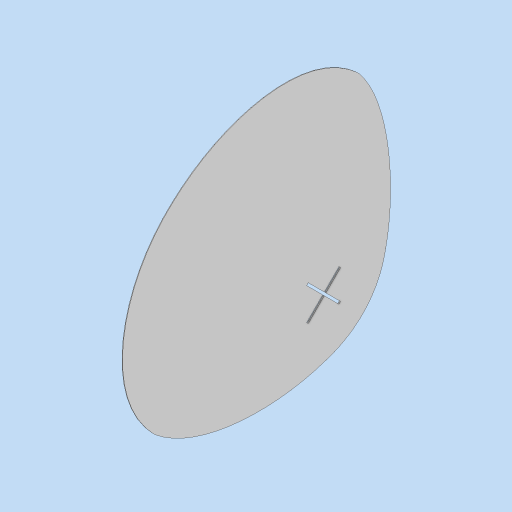
# Autodesk Inventor part: Sticker2
Saved by Autodesk Inventor 2024 (Build 280153000, 153)
## iProperties
Created: 2025-01-25
Part Number: Sticker2
Material: Generic
Document SubType Name: Modeling
Designer: Dmitry
Density: 1 g/cm^3
Appearance: Default
Author: Dmitry
Autodesk Inventor part; units mm, degrees
(part 1 of 3)
ref_plane "YZ Plane" through (0, 0, 0) normal (1, 0, 0) x (0, 1, 0)
ref_plane "XZ Plane" through (0, 0, 0) normal (0, 1, 0) x (-1, 0, 0)
ref_plane "XY Plane" through (0, 0, 0) normal (0, 0, 1) x (1, 0, 0)
sketch "Sketch1" plane through (0, 0, 0) normal (1, 0, 0) x (0, 1, 0)
  line L0 (-21.709644, 35.632021) -> (-25.631404, 35.976699)
  line L1 (-25.631404, 35.976699) -> (-30.886664, 35.950283)
  line L2 (-30.886664, 35.950283) -> (-36.111444, 35.341191)
  line L3 (-59.007004, 23.466691) -> (-59.883304, 22.478631)
  line L4 (-66.774324, 9.489325) -> (-68.001144, 5.643003)
  line L5 (-68.346584, 4.343793) -> (-69.034924, 1.649615)
  line L6 (-69.034924, 1.649615) -> (-70.464944, -6.596495)
  line L7 (-70.464944, -6.596495) -> (-71.331084, -17.731347)
  line L8 (-63.947304, -55.443921) -> (-61.640984, -58.857325)
  line L9 (-61.640984, -58.857325) -> (-60.729124, -59.867433)
  line L10 (-60.729124, -59.867433) -> (-59.807104, -60.803118)
  line L11 (-59.807104, -60.803118) -> (-56.515264, -63.098922)
  line L12 (-56.515264, -63.098922) -> (-51.475904, -65.518755)
  line L13 (-51.475904, -65.518755) -> (-46.101264, -67.289516)
  line L14 (-46.101264, -67.289516) -> (-42.187124, -68.287253)
  line L15 (-42.187124, -68.287253) -> (-40.871404, -68.578007)
  line L16 (-40.871404, -68.578007) -> (-38.123124, -69.126469)
  line L17 (-29.769064, -70.227534) -> (-18.534644, -70.775971)
  line L18 (-18.534644, -70.775971) -> (-7.300224, -70.206858)
  line L19 (1.048756, -69.074094) -> (3.794496, -68.507751)
  line L20 (3.794496, -68.507751) -> (5.293096, -68.172852)
  line L21 (5.293096, -68.172852) -> (9.755876, -66.987764)
  line L22 (9.755876, -66.987764) -> (15.577556, -64.968921)
  line L23 (15.577556, -64.968921) -> (21.069036, -62.265193)
  line L24 (26.042356, -58.690574) -> (27.380936, -57.473762)
  line L25 (27.380936, -57.473762) -> (30.792156, -53.170164)
  line L26 (30.792156, -53.170164) -> (34.183056, -46.747037)
  line L27 (37.050716, -34.324151) -> (37.106596, -32.509067)
  line L28 (37.106596, -32.509067) -> (37.154856, -30.830635)
  line L29 (37.154856, -30.830635) -> (36.888156, -25.784417)
  line L30 (36.888156, -25.784417) -> (35.856916, -19.170003)
  line L31 (31.632896, -6.464161) -> (28.567116, -0.472809)
  line L32 (28.567116, -0.472809) -> (24.942536, 5.211965)
  line L33 (24.942536, 5.211965) -> (20.832816, 10.540631)
  line L34 (16.298916, 15.461627) -> (15.361656, 16.394569)
  line L35 (15.361656, 16.394569) -> (12.438116, 19.080365)
  line L36 (12.438116, 19.080365) -> (8.330936, 22.466185)
  line L37 (4.005316, 25.574891) -> (-0.528584, 28.363049)
  line L38 (-10.152644, 32.798905) -> (-15.214864, 34.358719)
  line L39 (-15.214864, 34.358719) -> (-19.106144, 35.221303)
  line L40 (-21.592804, 34.167203) -> (-22.852644, 34.373959)
  line L41 (-22.852644, 34.373959) -> (-26.672804, 34.708731)
  line L42 (-26.672804, 34.708731) -> (-31.793444, 34.684093)
  line L43 (-31.793444, 34.684093) -> (-36.881064, 34.091511)
  line L44 (-58.298344, 23.455515) -> (-59.177184, 22.525621)
  line L45 (-59.177184, 22.525621) -> (-60.033164, 21.563469)
  line L46 (-66.743844, 8.913253) -> (-67.937644, 5.167769)
  line L47 (-67.937644, 5.167769) -> (-68.275464, 3.902849)
  line L48 (-68.275464, 3.902849) -> (-68.943484, 1.278775)
  line L49 (-68.943484, 1.278775) -> (-70.337944, -6.753467)
  line L50 (-70.337944, -6.753467) -> (-71.183764, -17.599013)
  line L51 (-63.990484, -54.327693) -> (-61.745124, -57.651537)
  line L52 (-61.745124, -57.651537) -> (-60.858664, -58.635456)
  line L53 (-60.858664, -58.635456) -> (-59.959504, -59.547723)
  line L54 (-59.959504, -59.547723) -> (-56.751484, -61.784294)
  line L55 (-56.751484, -61.784294) -> (-51.844204, -64.140703)
  line L56 (-51.844204, -64.140703) -> (-46.609264, -65.864652)
  line L57 (-46.609264, -65.864652) -> (-42.796724, -66.837548)
  line L58 (-42.796724, -66.837548) -> (-41.516564, -67.120047)
  line L59 (-41.516564, -67.120047) -> (-38.839404, -67.653345)
  line L60 (-30.701244, -68.726826) -> (-19.756384, -69.261521)
  line L61 (-19.756384, -69.261521) -> (-8.821684, -68.707547)
  line L62 (-0.686064, -67.603739) -> (1.988556, -67.051111)
  line L63 (1.988556, -67.051111) -> (3.449056, -66.724544)
  line L64 (3.449056, -66.724544) -> (7.789916, -65.571104)
  line L65 (7.789916, -65.571104) -> (13.459196, -63.606033)
  line L66 (13.459196, -63.606033) -> (18.810976, -60.972612)
  line L67 (24.957776, -56.305184) -> (28.280096, -52.113194)
  line L68 (34.376096, -33.757731) -> (34.431976, -31.990907)
  line L69 (34.431976, -31.990907) -> (34.482776, -30.356925)
  line L70 (34.482776, -30.356925) -> (34.218616, -25.442787)
  line L71 (34.218616, -25.442787) -> (33.215316, -18.998807)
  line L72 (15.318476, 13.582027) -> (14.165316, 14.729853)
  line L73 (14.165316, 14.729853) -> (13.250916, 15.639427)
  line L74 (13.250916, 15.639427) -> (10.401036, 18.254865)
  line L75 (10.401036, 18.254865) -> (6.405616, 21.551277)
  line L76 (2.191756, 24.578703) -> (-2.225304, 27.294725)
  line L77 (34.431976, -31.990907) -> (34.376096, -33.757731)
  line L78 (28.280096, -52.113194) -> (24.957776, -56.305184)
  line L79 (18.810976, -60.972612) -> (13.459196, -63.606033)
  line L80 (13.459196, -63.606033) -> (7.789916, -65.571104)
  line L81 (7.789916, -65.571104) -> (3.449056, -66.724544)
  line L82 (3.449056, -66.724544) -> (1.988556, -67.051111)
  line L83 (1.988556, -67.051111) -> (-0.686064, -67.603739)
  line L84 (-8.821684, -68.707547) -> (-19.756384, -69.261521)
  line L85 (-19.756384, -69.261521) -> (-30.701244, -68.726826)
  line L86 (-38.839404, -67.653345) -> (-41.516564, -67.120047)
  line L87 (-41.516564, -67.120047) -> (-42.796724, -66.837548)
  line L88 (-42.796724, -66.837548) -> (-46.609264, -65.864652)
  line L89 (-46.609264, -65.864652) -> (-51.844204, -64.140703)
  line L90 (-51.844204, -64.140703) -> (-56.748944, -61.784294)
  line L91 (-56.748944, -61.784294) -> (-59.956964, -59.547723)
  line L92 (-59.956964, -59.547723) -> (-60.856124, -58.635456)
  line L93 (-60.856124, -58.635456) -> (-61.745124, -57.651537)
  line L94 (-61.745124, -57.651537) -> (-63.990484, -54.327693)
  line L95 (-71.183764, -17.599013) -> (-70.337944, -6.753467)
  line L96 (-70.337944, -6.753467) -> (-68.943484, 1.278775)
  line L97 (-68.943484, 1.278775) -> (-68.275464, 3.902849)
  line L98 (-68.275464, 3.902849) -> (-67.937644, 5.167769)
  line L99 (-67.937644, 5.167769) -> (-66.743844, 8.913253)
  line L100 (-60.033164, 21.563469) -> (-59.177184, 22.525621)
  line L101 (-59.177184, 22.525621) -> (-58.298344, 23.455515)
  line L102 (-36.881064, 34.091511) -> (-31.793444, 34.684093)
  line L103 (-31.793444, 34.684093) -> (-26.672804, 34.708731)
  line L104 (-26.672804, 34.708731) -> (-22.852644, 34.373959)
  line L105 (-22.852644, 34.373959) -> (-21.592804, 34.167203)
  line L106 (-2.225304, 27.294725) -> (2.191756, 24.578703)
  line L107 (6.408156, 21.551277) -> (10.406116, 18.254865)
  line L108 (10.406116, 18.254865) -> (13.255996, 15.639427)
  line L109 (13.255996, 15.639427) -> (14.170396, 14.729853)
  line L110 (14.170396, 14.729853) -> (15.318476, 13.582027)
  line L111 (33.215316, -18.998807) -> (34.218616, -25.442787)
  line L112 (34.218616, -25.442787) -> (34.482776, -30.356925)
  line L113 (34.482776, -30.356925) -> (34.431976, -31.990907)
  line L114 (34.429436, -31.990907) -> (34.373556, -33.759001)
  line L115 (28.280096, -52.114591) -> (24.957776, -56.305184)
  line L116 (18.810976, -60.97124) -> (13.464276, -63.604662)
  line L117 (13.464276, -63.604662) -> (7.789916, -65.571104)
  line L118 (7.789916, -65.571104) -> (3.449056, -66.725941)
  line L119 (3.449056, -66.725941) -> (1.988556, -67.052534)
  line L120 (1.988556, -67.052534) -> (-0.686064, -67.605111)
  line L121 (-8.821684, -68.707547) -> (-19.756384, -69.261521)
  line L122 (-19.756384, -69.261521) -> (-30.701244, -68.726826)
  line L123 (-38.839404, -67.654717) -> (-41.516564, -67.120047)
  line L124 (-41.516564, -67.120047) -> (-42.796724, -66.837548)
  line L125 (-42.796724, -66.837548) -> (-46.606724, -65.864652)
  line L126 (-46.606724, -65.864652) -> (-51.841664, -64.140703)
  line L127 (-51.841664, -64.140703) -> (-56.748944, -61.784294)
  line L128 (-56.748944, -61.784294) -> (-59.956964, -59.547723)
  line L129 (-59.956964, -59.547723) -> (-60.858664, -58.635456)
  line L130 (-60.858664, -58.635456) -> (-61.745124, -57.651537)
  line L131 (-61.745124, -57.651537) -> (-63.990484, -54.327693)
  line L132 (-71.183764, -17.599013) -> (-70.337944, -6.752197)
  line L133 (-70.337944, -6.752197) -> (-68.943484, 1.278775)
  line L134 (-68.943484, 1.278775) -> (-68.275464, 3.902849)
  line L135 (-68.275464, 3.902849) -> (-67.937644, 5.167769)
  line L136 (-67.937644, 5.167769) -> (-66.743844, 8.913253)
  line L137 (-60.033164, 21.564993) -> (-59.177184, 22.526891)
  line L138 (-59.177184, 22.526891) -> (-58.298344, 23.457039)
  line L139 (-36.881064, 34.091511) -> (-31.793444, 34.684093)
  line L140 (-31.793444, 34.684093) -> (-26.672804, 34.708731)
  line L141 (-26.672804, 34.708731) -> (-22.852644, 34.373959)
  line L142 (-22.852644, 34.373959) -> (-21.592804, 34.167203)
  line L143 (-2.220224, 27.294725) -> (2.191756, 24.580227)
  line L144 (6.408156, 21.551277) -> (10.406116, 18.254865)
  line L145 (10.406116, 18.254865) -> (13.255996, 15.639427)
  line L146 (13.255996, 15.639427) -> (14.170396, 14.729853)
  line L147 (14.170396, 14.729853) -> (15.318476, 13.582027)
  line L148 (33.215316, -19.000331) -> (34.218616, -25.442787)
  line L149 (34.218616, -25.442787) -> (34.477696, -30.356925)
  line L150 (34.477696, -30.356925) -> (34.429436, -31.990907)
  line L151 (7.358116, -65.695158) -> (7.081256, -65.777835)
  line L152 (7.081256, -65.777835) -> (4.386316, -66.506815)
  line L153 (4.386316, -66.506815) -> (4.119616, -66.571585)
  line L154 (4.119616, -66.571585) -> (3.824976, -66.640495)
  line L155 (3.824976, -66.640495) -> (2.918196, -66.687333)
  line L156 (2.918196, -66.687333) -> (1.803136, -66.483396)
  line L157 (1.803136, -66.483396) -> (0.812536, -66.003819)
  line L158 (0.812536, -66.003819) -> (-0.015504, -65.294143)
  line L159 (-0.015504, -65.294143) -> (-0.647964, -64.39704)
  line L160 (-0.647964, -64.39704) -> (-1.031504, -63.358002)
  line L161 (-1.031504, -63.358002) -> (-1.140724, -62.22247)
  line L162 (-1.140724, -62.22247) -> (-1.021344, -61.318484)
  line L163 (-1.021344, -61.318484) -> (-0.929904, -61.034639)
  line L164 (-0.929904, -61.034639) -> (-0.820684, -60.695625)
  line L165 (-0.820684, -60.695625) -> (-0.439684, -58.935862)
  line L166 (-0.439684, -58.935862) -> (-0.287284, -57.101703)
  line L167 (-0.287284, -57.101703) -> (-0.294904, -56.726875)
  line L168 (-0.294904, -56.726875) -> (-0.305064, -55.986871)
  line L169 (-0.305064, -55.986871) -> (-0.678444, -53.775116)
  line L170 (-0.678444, -53.775116) -> (-1.676664, -51.086627)
  line L171 (-1.676664, -51.086627) -> (-3.208284, -48.720363)
  line L172 (-3.208284, -48.720363) -> (-5.194564, -46.734591)
  line L173 (-5.194564, -46.734591) -> (-7.549144, -45.190017)
  line L174 (-7.549144, -45.190017) -> (-10.198364, -44.146839)
  line L175 (-10.198364, -44.146839) -> (-13.055864, -43.661699)
  line L176 (-13.055864, -43.661699) -> (-15.308844, -43.683797)
  line L177 (-15.308844, -43.683797) -> (-16.042904, -43.796827)
  line L178 (-16.042904, -43.796827) -> (-16.268964, -43.831117)
  line L179 (-16.268964, -43.831117) -> (-18.295884, -44.302541)
  line L180 (-18.295884, -44.302541) -> (-18.481304, -44.361723)
  line L181 (-18.481304, -44.361723) -> (-18.712444, -44.434875)
  line L182 (-18.712444, -44.434875) -> (-19.438884, -44.556033)
  line L183 (-19.438884, -44.556033) -> (-20.378684, -44.539523)
  line L184 (-20.378684, -44.539523) -> (-21.275304, -44.324639)
  line L185 (-21.275304, -44.324639) -> (-22.095724, -43.931701)
  line L186 (-22.095724, -43.931701) -> (-22.817084, -43.375187)
  line L187 (-22.817084, -43.375187) -> (-23.406364, -42.672369)
  line L188 (-23.406364, -42.672369) -> (-23.835624, -41.840011)
  line L189 (-23.835624, -41.840011) -> (-24.051524, -41.134145)
  line L190 (-24.051524, -41.134145) -> (-24.082004, -40.894623)
  line L191 (-24.082004, -40.894623) -> (-24.209004, -40.036103)
  line L192 (-24.209004, -40.036103) -> (-24.854164, -37.500675)
  line L193 (-24.854164, -37.500675) -> (-26.147024, -34.259381)
  line L194 (-26.147024, -34.259381) -> (-27.955504, -31.241353)
  line L195 (-27.955504, -31.241353) -> (-29.631904, -29.148139)
  line L196 (-29.631904, -29.148139) -> (-30.259284, -28.521013)
  line L197 (-30.259284, -28.521013) -> (-31.021284, -27.757489)
  line L198 (-31.021284, -27.757489) -> (-33.607004, -25.767907)
  line L199 (-33.607004, -25.767907) -> (-37.376364, -23.753179)
  line L200 (-37.376364, -23.753179) -> (-41.463224, -22.514167)
  line L201 (-41.463224, -22.514167) -> (-44.699184, -22.094051)
  line L202 (-44.699184, -22.094051) -> (-45.778684, -22.094051)
  line L203 (-45.778684, -22.094051) -> (-46.916604, -22.094051)
  line L204 (-46.916604, -22.094051) -> (-50.335444, -22.565475)
  line L205 (-50.335444, -22.565475) -> (-53.980344, -23.662247)
  line L206 (-53.980344, -23.662247) -> (-54.686464, -23.975175)
  line L207 (-54.686464, -23.975175) -> (-55.402744, -24.282261)
  line L208 (-55.402744, -24.282261) -> (-57.719224, -24.823789)
  line L209 (-57.719224, -24.823789) -> (-60.711344, -24.846141)
  line L210 (-60.711344, -24.846141) -> (-63.533284, -24.125289)
  line L211 (-63.533284, -24.125289) -> (-66.070744, -22.747085)
  line L212 (-66.070744, -22.747085) -> (-68.199264, -20.800175)
  line L213 (-68.199264, -20.800175) -> (-69.799464, -18.366347)
  line L214 (-69.799464, -18.366347) -> (-70.746884, -15.536025)
  line L215 (-70.746884, -15.536025) -> (-70.985644, -13.168491)
  line L216 (-70.985644, -13.168491) -> (-70.927224, -12.391251)
  line L217 (-70.927224, -12.391251) -> (-70.805304, -10.869791)
  line L218 (-70.805304, -10.869791) -> (-70.274444, -6.318111)
  line L219 (-70.274444, -6.318111) -> (-69.258444, -0.307201)
  line L220 (-69.258444, -0.307201) -> (-67.795404, 5.604649)
  line L221 (-67.795404, 5.604649) -> (-66.380624, 9.963035)
  line L222 (-66.380624, 9.963035) -> (-65.816744, 11.379847)
  line L223 (-65.816744, 11.379847) -> (-65.814204, 11.387975)
  line L224 (-65.814204, 11.387975) -> (-65.788804, 11.460111)
  line L225 (-65.788804, 11.460111) -> (-65.786264, 11.466715)
  line L226 (-65.786264, 11.466715) -> (-65.623704, 11.930011)
  line L227 (-65.623704, 11.930011) -> (-64.597544, 13.127113)
  line L228 (-64.597544, 13.127113) -> (-62.817004, 13.871333)
  line L229 (-62.817004, 13.871333) -> (-60.906924, 13.634605)
  line L230 (-60.906924, 13.634605) -> (-59.606444, 12.751193)
  line L231 (-59.606444, 12.751193) -> (-59.329584, 12.347333)
  line L232 (-59.329584, 12.347333) -> (-58.885084, 11.698109)
  line L233 (-58.885084, 11.698109) -> (-57.236624, 9.963035)
  line L234 (-57.236624, 9.963035) -> (-54.635664, 8.138553)
  line L235 (-54.635664, 8.138553) -> (-51.625764, 6.972947)
  line L236 (-51.625764, 6.972947) -> (-49.141644, 6.560959)
  line L237 (-49.141644, 6.560959) -> (-48.313604, 6.560959)
  line L238 (-48.313604, 6.560959) -> (-48.222164, 6.560959)
  line L239 (-48.222164, 6.560959) -> (-47.975784, 6.566293)
  line L240 (-47.975784, 6.566293) -> (-47.945304, 6.566293)
  line L241 (-47.945304, 6.566293) -> (-47.196004, 6.587121)
  line L242 (-47.196004, 6.587121) -> (-43.571424, 7.422019)
  line L243 (-43.571424, 7.422019) -> (-40.302444, 9.184525)
  line L244 (-40.302444, 9.184525) -> (-39.730944, 9.669665)
  line L245 (-39.730944, 9.669665) -> (-39.141664, 10.168521)
  line L246 (-39.141664, 10.168521) -> (-37.597344, 11.928487)
  line L247 (-37.597344, 11.928487) -> (-36.065724, 14.539861)
  line L248 (-36.065724, 14.539861) -> (-35.174184, 17.415649)
  line L249 (-35.174184, 17.415649) -> (-34.920184, 19.703427)
  line L250 (-34.920184, 19.703427) -> (-34.948124, 20.461109)
  line L251 (-34.948124, 20.461109) -> (-34.976064, 21.142083)
  line L252 (-34.976064, 21.142083) -> (-35.682184, 24.350103)
  line L253 (-35.682184, 24.350103) -> (-37.071564, 27.224621)
  line L254 (-37.071564, 27.224621) -> (-37.442404, 27.737193)
  line L255 (-37.442404, 27.737193) -> (-37.759904, 28.180931)
  line L256 (-37.759904, 28.180931) -> (-38.222184, 29.862411)
  line L257 (-38.222184, 29.862411) -> (-37.836104, 31.969087)
  line L258 (-37.836104, 31.969087) -> (-36.482284, 33.643455)
  line L259 (-36.482284, 33.643455) -> (-34.904944, 34.409519)
  line L260 (-34.904944, 34.409519) -> (-34.358844, 34.468955)
  line L261 (-34.358844, 34.468955) -> (-34.229304, 34.483941)
  line L262 (-34.229304, 34.483941) -> (-32.905964, 34.602559)
  line L263 (-32.905964, 34.602559) -> (-32.771344, 34.610941)
  line L264 (-32.771344, 34.610941) -> (-32.192224, 34.645231)
  line L265 (-32.192224, 34.645231) -> (-26.421344, 34.584525)
  line L266 (-26.421344, 34.584525) -> (-25.847304, 34.540583)
  line L267 (-25.847304, 34.540583) -> (-25.324064, 34.500705)
  line L268 (-25.324064, 34.500705) -> (-23.789904, 33.829637)
  line L269 (-23.789904, 33.829637) -> (-22.418304, 32.292937)
  line L270 (-22.418304, 32.292937) -> (-21.905224, 30.288115)
  line L271 (-21.905224, 30.288115) -> (-22.192244, 28.632797)
  line L272 (-22.192244, 28.632797) -> (-22.446244, 28.167215)
  line L273 (-22.446244, 28.167215) -> (-22.453864, 28.157563)
  line L274 (-22.453864, 28.157563) -> (-22.509744, 28.050121)
  line L275 (-22.509744, 28.050121) -> (-22.512284, 28.039199)
  line L276 (-22.512284, 28.039199) -> (-22.931384, 27.252053)
  line L277 (-22.931384, 27.252053) -> (-24.026124, 23.047591)
  line L278 (-24.026124, 23.047591) -> (-23.756884, 18.711049)
  line L279 (-23.756884, 18.711049) -> (-23.497804, 17.856593)
  line L280 (-23.497804, 17.856593) -> (-23.307304, 17.229721)
  line L281 (-23.307304, 17.229721) -> (-22.484344, 15.418955)
  line L282 (-22.484344, 15.418955) -> (-21.039084, 13.258177)
  line L283 (-21.039084, 13.258177) -> (-19.192504, 11.424043)
  line L284 (-19.192504, 11.424043) -> (-17.574524, 10.270375)
  line L285 (-17.574524, 10.270375) -> (-16.992864, 9.961765)
  line L286 (-16.992864, 9.961765) -> (-16.512804, 9.705733)
  line L287 (-16.512804, 9.705733) -> (-13.949944, 8.793365)
  line L288 (-13.949944, 8.793365) -> (-11.531864, 8.392299)
  line L289 (-11.531864, 8.392299) -> (-10.726684, 8.392299)
  line L290 (-10.726684, 8.392299) -> (-9.822444, 8.392299)
  line L291 (-9.822444, 8.392299) -> (-7.117344, 8.885821)
  line L292 (-7.117344, 8.885821) -> (-3.833124, 10.298315)
  line L293 (-3.833124, 10.298315) -> (-1.041664, 12.530721)
  line L294 (-1.041664, 12.530721) -> (0.660136, 14.687181)
  line L295 (0.660136, 14.687181) -> (1.084316, 15.482455)
  line L296 (1.084316, 15.482455) -> (1.183376, 15.664319)
  line L297 (1.183376, 15.664319) -> (1.965696, 17.528933)
  line L298 (1.965696, 17.528933) -> (2.026656, 17.717655)
  line L299 (2.026656, 17.717655) -> (2.181596, 18.213463)
  line L300 (2.181596, 18.213463) -> (3.169656, 19.536549)
  line L301 (3.169656, 19.536549) -> (4.947656, 20.520291)
  line L302 (4.947656, 20.520291) -> (6.979656, 20.566011)
  line L303 (6.979656, 20.566011) -> (8.493496, 19.915263)
  line L304 (8.493496, 19.915263) -> (8.877036, 19.563981)
  line L305 (8.877036, 19.563981) -> (9.364716, 19.120243)
  line L306 (9.364716, 19.120243) -> (13.913856, 14.827643)
  line L307 (13.913856, 14.827643) -> (14.343116, 14.406003)
  line L308 (14.343116, 14.406003) -> (14.726656, 14.025765)
  line L309 (14.726656, 14.025765) -> (15.473416, 12.470015)
  line L310 (15.473416, 12.470015) -> (15.496276, 10.350639)
  line L311 (15.496276, 10.350639) -> (14.510756, 8.472309)
  line L312 (14.510756, 8.472309) -> (13.139156, 7.424813)
  line L313 (13.139156, 7.424813) -> (12.620996, 7.259459)
  line L314 (12.620996, 7.259459) -> (12.430496, 7.198753)
  line L315 (12.430496, 7.198753) -> (10.624556, 6.409321)
  line L316 (10.624556, 6.409321) -> (10.456916, 6.310261)
  line L317 (10.456916, 6.310261) -> (9.839696, 5.942215)
  line L318 (9.839696, 5.942215) -> (8.153136, 4.555883)
  line L319 (8.153136, 4.555883) -> (6.326876, 2.359291)
  line L320 (6.326876, 2.359291) -> (5.018776, -0.196711)
  line L321 (5.018776, -0.196711) -> (4.376156, -2.312531)
  line L322 (4.376156, -2.312531) -> (4.266936, -3.032875)
  line L323 (4.266936, -3.032875) -> (4.160256, -3.691751)
  line L324 (4.160256, -3.691751) -> (4.241536, -6.999085)
  line L325 (4.241536, -6.999085) -> (5.110216, -10.191611)
  line L326 (5.110216, -10.191611) -> (5.399776, -10.793845)
  line L327 (5.399776, -10.793845) -> (5.811256, -11.649825)
  line L328 (5.811256, -11.649825) -> (7.523216, -13.988403)
  line L329 (7.523216, -13.988403) -> (10.362936, -16.391751)
  line L330 (10.362936, -16.391751) -> (13.741136, -17.904829)
  line L331 (13.741136, -17.904829) -> (16.550376, -18.431117)
  line L332 (16.550376, -18.431117) -> (17.487636, -18.431117)
  line L333 (17.487636, -18.431117) -> (18.399496, -18.431117)
  line L334 (18.399496, -18.431117) -> (21.124916, -17.922863)
  line L335 (21.124916, -17.922863) -> (23.969716, -16.763607)
  line L336 (23.969716, -16.763607) -> (24.498036, -16.438487)
  line L337 (24.498036, -16.438487) -> (24.622496, -16.361525)
  line L338 (24.622496, -16.361525) -> (25.793436, -15.530437)
  line L339 (25.793436, -15.530437) -> (25.905196, -15.440775)
  line L340 (25.905196, -15.440775) -> (26.321756, -15.103209)
  line L341 (26.321756, -15.103209) -> (27.919416, -14.524597)
  line L342 (27.919416, -14.524597) -> (30.009836, -14.684363)
  line L343 (30.009836, -14.684363) -> (31.772596, -15.796375)
  line L344 (31.772596, -15.796375) -> (32.697156, -17.218267)
  line L345 (32.697156, -17.218267) -> (32.821616, -17.736681)
  line L346 (32.821616, -17.736681) -> (33.045136, -18.676481)
  line L347 (33.045136, -18.676481) -> (33.901116, -23.420947)
  line L348 (33.901116, -23.420947) -> (34.373556, -28.205545)
  line L349 (34.373556, -28.205545) -> (34.404036, -29.167697)
  line L350 (34.404036, -29.167697) -> (34.404036, -29.179889)
  line L351 (34.404036, -29.179889) -> (34.409116, -29.328987)
  line L352 (34.409116, -29.328987) -> (34.409116, -29.378263)
  line L353 (34.409116, -29.378263) -> (34.409116, -29.608641)
  line L354 (34.409116, -29.608641) -> (34.274496, -30.304347)
  line L355 (34.274496, -30.304347) -> (33.906196, -31.098097)
  line L356 (33.906196, -31.098097) -> (33.347396, -31.737669)
  line L357 (33.347396, -31.737669) -> (32.641276, -32.201981)
  line L358 (32.641276, -32.201981) -> (31.838636, -32.469189)
  line L359 (31.838636, -32.469189) -> (30.982656, -32.517703)
  line L360 (30.982656, -32.517703) -> (30.121596, -32.324663)
  line L361 (30.121596, -32.324663) -> (29.484056, -32.011735)
  line L362 (29.484056, -32.011735) -> (29.298636, -31.872289)
  line L363 (29.298636, -31.872289) -> (29.090356, -31.716841)
  line L364 (29.090356, -31.716841) -> (27.937196, -30.970081)
  line L365 (27.937196, -30.970081) -> (26.618936, -30.272597)
  line L366 (26.618936, -30.272597) -> (26.329376, -30.143057)
  line L367 (26.329376, -30.143057) -> (25.922976, -29.961447)
  line L368 (25.922976, -29.961447) -> (23.789376, -29.338385)
  line L369 (23.789376, -29.338385) -> (21.767536, -29.080575)
  line L370 (21.767536, -29.080575) -> (21.096976, -29.080575)
  line L371 (21.096976, -29.080575) -> (21.013156, -29.080575)
  line L372 (21.013156, -29.080575) -> (20.797256, -29.083369)
  line L373 (20.797256, -29.083369) -> (20.769316, -29.084639)
  line L374 (20.769316, -29.084639) -> (20.058116, -29.101403)
  line L375 (20.058116, -29.101403) -> (17.929596, -29.458273)
  line L376 (17.929596, -29.458273) -> (15.313396, -30.394009)
  line L377 (15.313396, -30.394009) -> (12.984216, -31.825807)
  line L378 (12.984216, -31.825807) -> (11.000476, -33.687373)
  line L379 (11.000476, -33.687373) -> (9.435836, -35.914445)
  line L380 (9.435836, -35.914445) -> (8.338556, -38.437681)
  line L381 (8.338556, -38.437681) -> (7.784836, -41.193581)
  line L382 (7.784836, -41.193581) -> (7.739116, -43.394491)
  line L383 (7.739116, -43.394491) -> (7.830556, -44.115089)
  line L384 (7.830556, -44.115089) -> (7.894056, -44.646965)
  line L385 (7.894056, -44.646965) -> (8.338556, -46.212367)
  line L386 (8.338556, -46.212367) -> (9.291056, -48.428263)
  line L387 (9.291056, -48.428263) -> (10.533116, -50.500903)
  line L388 (10.533116, -50.500903) -> (11.526256, -51.794881)
  line L389 (11.526256, -51.794881) -> (11.912336, -52.17522)
  line L390 (11.912336, -52.17522) -> (12.143476, -52.408088)
  line L391 (12.143476, -52.408088) -> (13.385536, -53.463661)
  line L392 (13.385536, -53.463661) -> (14.762216, -54.2726)
  line L393 (14.762216, -54.2726) -> (15.061936, -54.381464)
  line L394 (15.061936, -54.381464) -> (15.107656, -54.398)
  line L395 (15.107656, -54.398) -> (15.580096, -54.561982)
  line L396 (15.580096, -54.561982) -> (15.625816, -54.578518)
  line L397 (15.625816, -54.578518) -> (16.202396, -54.768662)
  line L398 (16.202396, -54.768662) -> (17.693376, -56.064037)
  line L399 (17.693376, -56.064037) -> (18.516336, -58.308863)
  line L400 (18.516336, -58.308863) -> (18.046436, -60.654274)
  line L401 (18.046436, -60.654274) -> (16.773896, -62.164609)
  line L402 (16.773896, -62.164609) -> (16.235416, -62.444364)
  line L403 (16.235416, -62.444364) -> (15.559776, -62.794351)
  line L404 (15.559776, -62.794351) -> (11.980916, -64.311594)
  line L405 (11.980916, -64.311594) -> (8.158216, -65.506334)
  line L406 (8.158216, -65.506334) -> (7.358116, -65.695158)
  line L407 (-14.849104, -68.58489) -> (-15.016744, -68.589031)
  line L408 (-15.016744, -68.589031) -> (-16.622024, -68.499445)
  line L409 (-16.622024, -68.499445) -> (-16.776964, -68.478769)
  line L410 (-16.776964, -68.478769) -> (-17.264644, -68.346486)
  line L411 (-17.264644, -68.346486) -> (-18.676884, -67.785629)
  line L412 (-18.676884, -67.785629) -> (-20.414244, -66.794825)
  line L413 (-20.414244, -66.794825) -> (-21.950944, -65.538059)
  line L414 (-21.950944, -65.538059) -> (-23.261584, -64.044259)
  line L415 (-23.261584, -64.044259) -> (-24.308064, -62.347895)
  line L416 (-24.308064, -62.347895) -> (-25.067524, -60.477871)
  line L417 (-25.067524, -60.477871) -> (-25.496784, -58.465962)
  line L418 (-25.496784, -58.465962) -> (-25.603464, -56.87295)
  line L419 (-25.603464, -56.87295) -> (-25.578064, -56.345164)
  line L420 (-25.578064, -56.345164) -> (-25.550124, -55.79533)
  line L421 (-25.550124, -55.79533) -> (-25.260564, -54.159595)
  line L422 (-25.260564, -54.159595) -> (-24.562064, -52.115962)
  line L423 (-24.562064, -52.115962) -> (-23.518124, -50.252745)
  line L424 (-23.518124, -50.252745) -> (-22.169384, -48.611651)
  line L425 (-22.169384, -48.611651) -> (-20.553944, -47.229383)
  line L426 (-20.553944, -47.229383) -> (-18.712444, -46.150391)
  line L427 (-18.712444, -46.150391) -> (-16.685524, -45.410489)
  line L428 (-16.685524, -45.410489) -> (-15.054844, -45.090703)
  line L429 (-15.054844, -45.090703) -> (-14.503664, -45.053619)
  line L430 (-14.503664, -45.053619) -> (-13.873744, -45.009423)
  line L431 (-13.873744, -45.009423) -> (-11.953504, -45.144551)
  line L432 (-11.953504, -45.144551) -> (-9.565904, -45.742467)
  line L433 (-9.565904, -45.742467) -> (-7.399284, -46.795297)
  line L434 (-7.399284, -46.795297) -> (-5.501904, -48.247923)
  line L435 (-5.501904, -48.247923) -> (-3.932184, -50.043449)
  line L436 (-3.932184, -50.043449) -> (-2.743464, -52.131126)
  line L437 (-2.743464, -52.131126) -> (-1.989084, -54.453118)
  line L438 (-1.989084, -54.453118) -> (-1.722384, -56.331372)
  line L439 (-1.722384, -56.331372) -> (-1.722384, -56.958396)
  line L440 (-1.722384, -56.958396) -> (-1.722384, -57.922986)
  line L441 (-1.722384, -57.922986) -> (-2.365004, -60.819653)
  line L442 (-2.365004, -60.819653) -> (-4.140464, -64.155867)
  line L443 (-4.140464, -64.155867) -> (-6.843024, -66.750731)
  line L444 (-6.843024, -66.750731) -> (-9.360164, -68.130129)
  line L445 (-9.360164, -68.130129) -> (-10.256784, -68.397489)
  line L446 (-10.256784, -68.397489) -> (-10.625084, -68.415371)
  line L447 (-10.625084, -68.415371) -> (-14.452864, -68.571098)
  line L448 (-14.452864, -68.571098) -> (-14.849104, -68.58489)
  line L449 (-60.167784, 21.241143) -> (-59.451504, 22.092805)
  line L450 (-46.781984, 31.156287) -> (-45.740584, 31.581991)
  line L451 (-45.740584, 31.581991) -> (-45.199564, 31.463627)
  line L452 (-45.199564, 31.463627) -> (-43.614604, 30.901271)
  line L453 (-43.614604, 30.901271) -> (-41.681664, 29.852505)
  line L454 (-41.681664, 29.852505) -> (-39.979864, 28.475825)
  line L455 (-39.979864, 28.475825) -> (-38.557464, 26.811109)
  line L456 (-38.557464, 26.811109) -> (-37.452564, 24.898489)
  line L457 (-37.452564, 24.898489) -> (-36.715964, 22.778859)
  line L458 (-36.715964, 22.778859) -> (-36.383224, 20.492859)
  line L459 (-36.383224, 20.492859) -> (-36.418784, 18.673965)
  line L460 (-36.418784, 18.673965) -> (-36.507684, 18.078589)
  line L461 (-36.507684, 18.078589) -> (-36.583884, 17.560683)
  line L462 (-36.583884, 17.560683) -> (-37.000444, 16.029571)
  line L463 (-37.000444, 16.029571) -> (-37.836104, 14.144383)
  line L464 (-37.836104, 14.144383) -> (-38.979104, 12.451981)
  line L465 (-38.979104, 12.451981) -> (-40.386264, 10.987163)
  line L466 (-40.386264, 10.987163) -> (-42.022024, 9.778631)
  line L467 (-42.022024, 9.778631) -> (-43.848284, 8.856865)
  line L468 (-43.848284, 8.856865) -> (-45.829484, 8.254631)
  line L469 (-45.829484, 8.254631) -> (-47.399204, 8.016125)
  line L470 (-47.399204, 8.016125) -> (-47.924984, 7.999615)
  line L471 (-47.924984, 7.999615) -> (-47.958004, 7.999615)
  line L472 (-47.958004, 7.999615) -> (-48.224704, 7.994027)
  line L473 (-48.224704, 7.994027) -> (-48.313604, 7.994027)
  line L474 (-48.313604, 7.994027) -> (-48.897804, 7.994027)
  line L475 (-48.897804, 7.994027) -> (-50.645324, 8.224405)
  line L476 (-50.645324, 8.224405) -> (-52.827184, 8.881503)
  line L477 (-52.827184, 8.881503) -> (-54.816004, 9.926205)
  line L478 (-54.816004, 9.926205) -> (-56.566064, 11.315077)
  line L479 (-56.566064, 11.315077) -> (-58.026564, 13.004431)
  line L480 (-58.026564, 13.004431) -> (-59.156864, 14.951849)
  line L481 (-59.156864, 14.951849) -> (-59.906164, 17.115421)
  line L482 (-59.906164, 17.115421) -> (-60.208424, 18.865481)
  line L483 (-60.208424, 18.865481) -> (-60.228744, 19.451205)
  line L484 (-60.228744, 19.451205) -> (-60.236364, 19.602843)
  line L485 (-60.236364, 19.602843) -> (-60.183024, 21.095093)
  line L486 (-60.183024, 21.095093) -> (-60.167784, 21.241143)
  line L487 (-0.178064, 16.154793) -> (-0.566684, 15.428861)
  line L488 (-0.566684, 15.428861) -> (-2.133864, 13.464933)
  line L489 (-2.133864, 13.464933) -> (-4.656084, 11.479161)
  line L490 (-4.656084, 11.479161) -> (-7.577084, 10.248531)
  line L491 (-7.577084, 10.248531) -> (-9.939284, 9.825621)
  line L492 (-9.939284, 9.825621) -> (-10.726684, 9.825621)
  line L493 (-10.726684, 9.825621) -> (-11.691884, 9.825621)
  line L494 (-11.691884, 9.825621) -> (-14.592564, 10.473321)
  line L495 (-14.592564, 10.473321) -> (-17.658344, 12.026277)
  line L496 (-17.658344, 12.026277) -> (-18.227304, 12.478143)
  line L497 (-18.227304, 12.478143) -> (-18.882624, 12.999097)
  line L498 (-18.882624, 12.999097) -> (-20.470124, 15.029065)
  line L499 (-20.470124, 15.029065) -> (-21.961104, 18.293727)
  line L500 (-21.961104, 18.293727) -> (-22.568164, 21.832455)
  line L501 (-22.568164, 21.832455) -> (-22.400524, 24.405221)
  line L502 (-22.400524, 24.405221) -> (-22.149064, 25.201765)
  line L503 (-22.149064, 25.201765) -> (-21.948404, 25.852005)
  line L504 (-21.948404, 25.852005) -> (-21.059404, 27.712555)
  line L505 (-21.059404, 27.712555) -> (-19.520164, 29.818215)
  line L506 (-19.520164, 29.818215) -> (-17.622784, 31.493853)
  line L507 (-17.622784, 31.493853) -> (-16.017504, 32.469213)
  line L508 (-16.017504, 32.469213) -> (-15.446004, 32.714831)
  line L509 (-15.446004, 32.714831) -> (-14.054084, 32.331799)
  line L510 (-0.724164, 26.513421) -> (0.530596, 25.749897)
  line L511 (0.530596, 25.749897) -> (0.731256, 25.183731)
  line L512 (0.731256, 25.183731) -> (1.104636, 23.399127)
  line L513 (1.104636, 23.399127) -> (1.193536, 20.965553)
  line L514 (1.193536, 20.965553) -> (0.774436, 18.525121)
  line L515 (0.774436, 18.525121) -> (0.119116, 16.715625)
  line L516 (0.119116, 16.715625) -> (-0.178064, 16.154793)
  line L517 (29.232596, -7.095351) -> (29.130996, -7.700379)
  line L518 (29.130996, -7.700379) -> (28.567116, -9.472537)
  line L519 (28.567116, -9.472537) -> (27.411416, -11.674717)
  line L520 (27.411416, -11.674717) -> (25.801056, -13.617563)
  line L521 (25.801056, -13.617563) -> (24.294836, -14.878673)
  line L522 (24.294836, -14.878673) -> (23.746196, -15.218779)
  line L523 (23.746196, -15.218779) -> (23.255976, -15.519261)
  line L524 (23.255976, -15.519261) -> (20.685496, -16.561169)
  line L525 (20.685496, -16.561169) -> (18.290276, -16.999319)
  line L526 (18.290276, -16.999319) -> (17.487636, -16.999319)
  line L527 (17.487636, -16.999319) -> (16.725636, -16.999319)
  line L528 (16.725636, -16.999319) -> (14.437096, -16.603841)
  line L529 (14.437096, -16.603841) -> (11.582136, -15.442045)
  line L530 (11.582136, -15.442045) -> (9.085316, -13.554317)
  line L531 (9.085316, -13.554317) -> (7.507976, -11.674717)
  line L532 (7.507976, -11.674717) -> (7.109196, -10.977487)
  line L533 (7.109196, -10.977487) -> (6.824716, -10.475837)
  line L534 (6.824716, -10.475837) -> (6.164316, -8.860651)
  line L535 (6.164316, -8.860651) -> (5.661396, -6.654407)
  line L536 (5.661396, -6.654407) -> (5.580116, -4.420731)
  line L537 (5.580116, -4.420731) -> (5.910316, -2.222869)
  line L538 (5.910316, -2.222869) -> (6.636756, -0.120003)
  line L539 (6.636756, -0.120003) -> (7.744196, 1.821827)
  line L540 (7.744196, 1.821827) -> (9.212316, 3.542931)
  line L541 (9.212316, 3.542931) -> (10.545816, 4.670183)
  line L542 (10.545816, 4.670183) -> (11.033496, 4.980063)
  line L543 (11.033496, 4.980063) -> (11.531336, 5.301627)
  line L544 (11.531336, 5.301627) -> (14.172936, 6.407797)
  line L545 (14.172936, 6.407797) -> (16.641816, 6.872363)
  line L546 (16.641816, 6.872363) -> (17.464776, 6.872363)
  line L547 (17.464776, 6.872363) -> (18.000716, 6.872363)
  line L548 (18.000716, 6.872363) -> (19.613616, 6.676783)
  line L549 (19.613616, 6.676783) -> (21.350976, 6.226187)
  line L550 (21.350976, 6.226187) -> (21.691336, 6.097663)
  line L551 (28.727136, -5.939397) -> (29.232596, -7.095351)
  line L552 (28.244536, -51.997446) -> (27.764476, -52.35711)
  line L553 (27.764476, -52.35711) -> (25.059376, -53.703462)
  line L554 (25.059376, -53.703462) -> (22.026616, -54.360789)
  line L555 (22.026616, -54.360789) -> (21.378916, -54.377324)
  line L556 (21.378916, -54.377324) -> (21.356056, -54.377324)
  line L557 (21.356056, -54.377324) -> (21.150316, -54.381464)
  line L558 (21.150316, -54.381464) -> (21.086816, -54.381464)
  line L559 (21.086816, -54.381464) -> (20.494996, -54.381464)
  line L560 (20.494996, -54.381464) -> (18.724616, -54.147175)
  line L561 (18.724616, -54.147175) -> (16.517356, -53.473338)
  line L562 (16.517356, -53.473338) -> (14.515836, -52.406716)
  line L563 (14.515836, -52.406716) -> (12.758156, -50.991377)
  line L564 (12.758156, -50.991377) -> (11.297656, -49.271797)
  line L565 (11.297656, -49.271797) -> (10.182596, -47.291359)
  line L566 (10.182596, -47.291359) -> (9.453616, -45.097561)
  line L567 (9.453616, -45.097561) -> (9.174216, -43.325403)
  line L568 (9.174216, -43.325403) -> (9.164056, -42.734345)
  line L569 (9.164056, -42.734345) -> (9.146276, -42.133381)
  line L570 (9.146276, -42.133381) -> (9.346936, -40.324139)
  line L571 (9.346936, -40.324139) -> (9.984476, -38.066841)
  line L572 (9.984476, -38.066841) -> (11.036036, -36.015029)
  line L573 (11.036036, -36.015029) -> (12.450816, -34.213661)
  line L574 (12.450816, -34.213661) -> (14.183096, -32.714553)
  line L575 (14.183096, -32.714553) -> (16.184616, -31.565203)
  line L576 (16.184616, -31.565203) -> (18.407116, -30.815395)
  line L577 (18.407116, -30.815395) -> (20.202896, -30.530407)
  line L578 (20.202896, -30.530407) -> (20.804876, -30.516691)
  line L579 (20.804876, -30.516691) -> (20.830276, -30.515167)
  line L580 (20.830276, -30.515167) -> (21.030936, -30.512373)
  line L581 (21.030936, -30.512373) -> (21.096976, -30.512373)
  line L582 (21.096976, -30.512373) -> (21.676096, -30.512373)
  line L583 (21.676096, -30.512373) -> (23.418536, -30.738687)
  line L584 (23.418536, -30.738687) -> (25.592776, -31.390197)
  line L585 (25.592776, -31.390197) -> (27.571436, -32.425247)
  line L586 (27.571436, -32.425247) -> (29.313876, -33.798879)
  line L587 (29.313876, -33.798879) -> (30.774376, -35.470707)
  line L588 (30.774376, -35.470707) -> (31.902136, -37.397297)
  line L589 (31.902136, -37.397297) -> (32.664136, -39.535723)
  line L590 (32.664136, -39.535723) -> (32.979096, -41.263939)
  line L591 (32.979096, -41.263939) -> (33.007036, -41.844075)
  line L592 (33.007036, -41.844075) -> (32.745416, -42.772953)
  line L593 (28.770316, -51.23951) -> (28.244536, -51.997446)
  line L594 (20.599136, 20.910435) -> (19.661876, 21.984093)
  line L595 (19.661876, 21.984093) -> (16.629116, 25.015583)
  line L596 (16.629116, 25.015583) -> (12.257776, 28.747097)
  line L597 (12.257776, 28.747097) -> (7.535916, 32.082371)
  line L598 (7.535916, 32.082371) -> (2.519416, 34.996513)
  line L599 (2.519416, 34.996513) -> (-2.738384, 37.468949)
  line L600 (-2.738384, 37.468949) -> (-8.194304, 39.472755)
  line L601 (-8.194304, 39.472755) -> (-13.782304, 40.987103)
  line L602 (-13.782304, 40.987103) -> (-19.456664, 41.986085)
  line L603 (-19.456664, 41.986085) -> (-25.166584, 42.447603)
  line L604 (-25.166584, 42.447603) -> (-30.851104, 42.347019)
  line L605 (-30.851104, 42.347019) -> (-36.469584, 41.662235)
  line L606 (-36.469584, 41.662235) -> (-41.958524, 40.369883)
  line L607 (-41.958524, 40.369883) -> (-47.272204, 38.443293)
  line L608 (-47.272204, 38.443293) -> (-52.354744, 35.861891)
  line L609 (-52.354744, 35.861891) -> (-57.155344, 32.600277)
  line L610 (-57.155344, 32.600277) -> (-60.571644, 29.694009)
  line L611 (-60.571644, 29.694009) -> (-61.618124, 28.635591)
  line L612 (-61.618124, 28.635591) -> (-62.369964, 27.748115)
  line L613 (-62.369964, 27.748115) -> (-64.437524, 24.924905)
  line L614 (-64.437524, 24.924905) -> (-66.926724, 20.862175)
  line L615 (-66.926724, 20.862175) -> (-69.085724, 16.492359)
  line L616 (-69.085724, 16.492359) -> (-70.922144, 11.855589)
  line L617 (-70.922144, 11.855589) -> (-72.438524, 6.993521)
  line L618 (-72.438524, 6.993521) -> (-73.637404, 1.946033)
  line L619 (-73.637404, 1.946033) -> (-74.521324, -3.242425)
  line L620 (-74.521324, -3.242425) -> (-75.095364, -8.532737)
  line L621 (-75.095364, -8.532737) -> (-75.362064, -13.882231)
  line L622 (-75.362064, -13.882231) -> (-75.329044, -19.251029)
  line L623 (-75.329044, -19.251029) -> (-74.993764, -24.596459)
  line L624 (-74.993764, -24.596459) -> (-74.363844, -29.878389)
  line L625 (-74.363844, -29.878389) -> (-73.441824, -35.053131)
  line L626 (-73.441824, -35.053131) -> (-72.230244, -40.081569)
  line L627 (-72.230244, -40.081569) -> (-70.731644, -44.921285)
  line L628 (-70.731644, -44.921285) -> (-69.441324, -48.395243)
  line L629 (-69.441324, -48.395243) -> (-68.953644, -49.530877)
  line L630 (-68.953644, -49.530877) -> (-68.570104, -50.426481)
  line L631 (-68.570104, -50.426481) -> (-67.221364, -53.028203)
  line L632 (-67.221364, -53.028203) -> (-65.128404, -56.283137)
  line L633 (-65.128404, -56.283137) -> (-62.702704, -59.270736)
  line L634 (-62.702704, -59.270736) -> (-59.969664, -61.964812)
  line L635 (-59.969664, -61.964812) -> (-56.959764, -64.341922)
  line L636 (-56.959764, -64.341922) -> (-53.695864, -66.375903)
  line L637 (-53.695864, -66.375903) -> (-50.208444, -68.044709)
  line L638 (-50.208444, -68.044709) -> (-47.455084, -69.056162)
  line L639 (-47.455084, -69.056162) -> (-46.517824, -69.322125)
  line L640 (-46.517824, -69.322125) -> (-45.420544, -69.633606)
  line L641 (-45.420544, -69.633606) -> (-42.082984, -70.421793)
  line L642 (-42.082984, -70.421793) -> (-37.378904, -71.292734)
  line L643 (-37.378904, -71.292734) -> (-32.453844, -71.932153)
  line L644 (-32.453844, -71.932153) -> (-27.361144, -72.340026)
  line L645 (-27.361144, -72.340026) -> (-22.146524, -72.515058)
  line L646 (-22.146524, -72.515058) -> (-16.860784, -72.457197)
  line L647 (-16.860784, -72.457197) -> (-11.554724, -72.16502)
  line L648 (-11.554724, -72.16502) -> (-6.284224, -71.638631)
  line L649 (-6.284224, -71.638631) -> (-1.092464, -70.875183)
  line L650 (-1.092464, -70.875183) -> (3.969756, -69.877496)
  line L651 (3.969756, -69.877496) -> (8.849096, -68.641405)
  line L652 (8.849096, -68.641405) -> (13.494756, -67.168282)
  line L653 (13.494756, -67.168282) -> (17.863556, -65.455356)
  line L654 (17.863556, -65.455356) -> (21.894536, -63.504078)
  line L655 (21.894536, -63.504078) -> (25.547056, -61.312972)
  line L656 (25.547056, -61.312972) -> (28.000696, -59.535328)
  line L657 (28.000696, -59.535328) -> (28.767776, -58.882116)
  line L658 (28.767776, -58.882116) -> (29.755836, -57.854102)
  line L659 (29.755836, -57.854102) -> (32.450776, -54.506864)
  line L660 (32.450776, -54.506864) -> (35.420036, -49.840757)
  line L661 (35.420036, -49.840757) -> (37.706036, -44.926619)
  line L662 (37.706036, -44.926619) -> (39.346876, -39.811313)
  line L663 (39.346876, -39.811313) -> (40.370496, -34.537511)
  line L664 (40.370496, -34.537511) -> (40.814996, -29.152457)
  line L665 (40.814996, -29.152457) -> (40.713396, -23.700601)
  line L666 (40.713396, -23.700601) -> (40.091096, -18.228679)
  line L667 (40.091096, -18.228679) -> (38.991276, -12.778347)
  line L668 (38.991276, -12.778347) -> (37.441876, -7.398373)
  line L669 (37.441876, -7.398373) -> (35.475916, -2.131937)
  line L670 (35.475916, -2.131937) -> (33.131496, 2.976765)
  line L671 (33.131496, 2.976765) -> (30.439096, 7.879727)
  line L672 (30.439096, 7.879727) -> (27.429196, 12.533515)
  line L673 (27.429196, 12.533515) -> (24.139896, 16.892155)
  line L674 (24.139896, 16.892155) -> (21.521156, 19.942949)
  line L675 (21.521156, 19.942949) -> (20.599136, 20.910435)
  line L676 (-13.657844, -68.892205) -> (-13.058404, -68.892205)
  line L677 (-13.058404, -68.892205) -> (-11.255004, -68.64966)
  line L678 (-11.255004, -68.64966) -> (-9.014724, -67.953726)
  line L679 (-9.014724, -67.953726) -> (-6.987804, -66.854084)
  line L680 (-6.987804, -66.854084) -> (-5.219964, -65.396098)
  line L681 (-5.219964, -65.396098) -> (-3.762004, -63.629452)
  line L682 (-3.762004, -63.629452) -> (-2.662184, -61.602354)
  line L683 (-2.662184, -61.602354) -> (-1.966224, -59.363065)
  line L684 (-1.966224, -59.363065) -> (-1.722384, -57.559208)
  line L685 (-1.722384, -57.559208) -> (-1.722384, -56.958396)
  line L686 (-1.722384, -56.958396) -> (-1.722384, -56.356162)
  line L687 (-1.722384, -56.356162) -> (-1.966224, -54.552356)
  line L688 (-1.966224, -54.552356) -> (-2.662184, -52.313015)
  line L689 (-2.662184, -52.313015) -> (-3.762004, -50.286019)
  line L690 (-3.762004, -50.286019) -> (-5.219964, -48.519195)
  line L691 (-5.219964, -48.519195) -> (-6.987804, -47.061235)
  line L692 (-6.987804, -47.061235) -> (-9.014724, -45.961669)
  line L693 (-9.014724, -45.961669) -> (-11.255004, -45.265709)
  line L694 (-11.255004, -45.265709) -> (-13.058404, -45.024663)
  line L695 (-13.058404, -45.024663) -> (-13.657844, -45.024663)
  line L696 (-13.657844, -45.024663) -> (-14.262364, -45.024663)
  line L697 (-14.262364, -45.024663) -> (-16.063224, -45.265709)
  line L698 (-16.063224, -45.265709) -> (-18.303504, -45.961669)
  line L699 (-18.303504, -45.961669) -> (-20.332964, -47.061235)
  line L700 (-20.332964, -47.061235) -> (-22.095724, -48.519195)
  line L701 (-22.095724, -48.519195) -> (-23.556224, -50.286019)
  line L702 (-23.556224, -50.286019) -> (-24.653504, -52.313015)
  line L703 (-24.653504, -52.313015) -> (-25.352004, -54.552356)
  line L704 (-25.352004, -54.552356) -> (-25.593304, -56.356162)
  line L705 (-25.593304, -56.356162) -> (-25.593304, -56.958396)
  line L706 (-25.593304, -56.958396) -> (-25.593304, -57.559208)
  line L707 (-25.593304, -57.559208) -> (-25.352004, -59.363065)
  line L708 (-25.352004, -59.363065) -> (-24.653504, -61.602354)
  line L709 (-24.653504, -61.602354) -> (-23.556224, -63.629452)
  line L710 (-23.556224, -63.629452) -> (-22.095724, -65.396098)
  line L711 (-22.095724, -65.396098) -> (-20.332964, -66.854084)
  line L712 (-20.332964, -66.854084) -> (-18.303504, -67.953726)
  line L713 (-18.303504, -67.953726) -> (-16.063224, -68.64966)
  line L714 (-16.063224, -68.64966) -> (-14.262364, -68.892205)
  line L715 (-14.262364, -68.892205) -> (-13.657844, -68.892205)
  line L716 (-47.828464, 8.003933) -> (-47.229024, 8.028571)
  line L717 (-47.229024, 8.028571) -> (-45.435784, 8.342769)
  line L718 (-45.435784, 8.342769) -> (-43.223444, 9.126613)
  line L719 (-43.223444, 9.126613) -> (-41.242244, 10.306443)
  line L720 (-41.242244, 10.306443) -> (-39.537904, 11.833237)
  line L721 (-39.537904, 11.833237) -> (-38.151064, 13.654925)
  line L722 (-38.151064, 13.654925) -> (-37.132524, 15.724771)
  line L723 (-37.132524, 15.724771) -> (-36.528004, 17.991721)
  line L724 (-36.528004, 17.991721) -> (-36.355284, 19.804011)
  line L725 (-36.355284, 19.804011) -> (-36.380684, 20.403197)
  line L726 (-36.380684, 20.403197) -> (-36.406084, 21.004161)
  line L727 (-36.406084, 21.004161) -> (-36.718504, 22.796893)
  line L728 (-36.718504, 22.796893) -> (-37.503364, 25.008725)
  line L729 (-37.503364, 25.008725) -> (-38.684464, 26.990433)
  line L730 (-38.684464, 26.990433) -> (-40.208464, 28.696297)
  line L731 (-40.208464, 28.696297) -> (-42.032184, 30.082883)
  line L732 (-42.032184, 30.082883) -> (-44.102284, 31.100915)
  line L733 (-44.102284, 31.100915) -> (-46.370504, 31.705943)
  line L734 (-46.370504, 31.705943) -> (-48.181524, 31.876885)
  line L735 (-48.181524, 31.876885) -> (-48.780964, 31.851993)
  line L736 (-48.780964, 31.851993) -> (-49.380404, 31.828625)
  line L737 (-49.380404, 31.828625) -> (-51.173644, 31.514427)
  line L738 (-51.173644, 31.514427) -> (-53.383444, 30.730583)
  line L739 (-53.383444, 30.730583) -> (-55.367184, 29.550753)
  line L740 (-55.367184, 29.550753) -> (-57.074064, 28.023959)
  line L741 (-57.074064, 28.023959) -> (-58.458364, 26.200747)
  line L742 (-58.458364, 26.200747) -> (-59.479444, 24.131155)
  line L743 (-59.479444, 24.131155) -> (-60.083964, 21.865475)
  line L744 (-60.083964, 21.865475) -> (-60.254144, 20.053185)
  line L745 (-60.254144, 20.053185) -> (-60.228744, 19.451205)
  line L746 (-60.228744, 19.451205) -> (-60.205884, 18.851765)
  line L747 (-60.205884, 18.851765) -> (-59.890924, 17.059033)
  line L748 (-59.890924, 17.059033) -> (-59.108604, 14.848471)
  line L749 (-59.108604, 14.848471) -> (-57.927504, 12.866763)
  line L750 (-57.927504, 12.866763) -> (-56.400964, 11.159375)
  line L751 (-56.400964, 11.159375) -> (-54.577244, 9.774313)
  line L752 (-54.577244, 9.774313) -> (-52.507144, 8.756027)
  line L753 (-52.507144, 8.756027) -> (-50.241464, 8.151253)
  line L754 (-50.241464, 8.151253) -> (-48.430444, 7.980311)
  line L755 (-48.430444, 7.980311) -> (-47.828464, 8.003933)
  line L756 (-16.317224, 11.225415) -> (-15.788904, 10.944491)
  line L757 (-15.788904, 10.944491) -> (-14.084564, 10.310761)
  line L758 (-14.084564, 10.310761) -> (-11.778244, 9.872611)
  line L759 (-11.778244, 9.872611) -> (-9.474464, 9.891661)
  line L760 (-9.474464, 9.891661) -> (-7.229104, 10.347591)
  line L761 (-7.229104, 10.347591) -> (-5.113284, 11.222875)
  line L762 (-5.113284, 11.222875) -> (-3.190504, 12.494653)
  line L763 (-3.190504, 12.494653) -> (-1.521724, 14.145653)
  line L764 (-1.521724, 14.145653) -> (-0.460004, 15.624187)
  line L765 (-0.460004, 15.624187) -> (-0.178064, 16.154793)
  line L766 (-0.178064, 16.154793) -> (0.103876, 16.686669)
  line L767 (0.103876, 16.686669) -> (0.736336, 18.392787)
  line L768 (0.736336, 18.392787) -> (1.173216, 20.696821)
  line L769 (1.173216, 20.696821) -> (1.155436, 23.003649)
  line L770 (1.155436, 23.003649) -> (0.700776, 25.247231)
  line L771 (0.700776, 25.247231) -> (-0.175524, 27.363813)
  line L772 (-0.175524, 27.363813) -> (-1.448064, 29.287609)
  line L773 (-1.448064, 29.287609) -> (-3.099064, 30.953341)
  line L774 (-3.099064, 30.953341) -> (-4.577344, 32.016077)
  line L775 (-4.577344, 32.016077) -> (-5.105664, 32.297255)
  line L776 (-5.105664, 32.297255) -> (-5.639064, 32.579703)
  line L777 (-5.639064, 32.579703) -> (-7.345944, 33.213687)
  line L778 (-7.345944, 33.213687) -> (-9.649724, 33.651837)
  line L779 (-9.649724, 33.651837) -> (-11.958584, 33.632533)
  line L780 (-11.958584, 33.632533) -> (-14.201404, 33.174825)
  line L781 (-14.201404, 33.174825) -> (-16.317224, 32.301319)
  line L782 (-16.317224, 32.301319) -> (-18.240004, 31.027763)
  line L783 (-18.240004, 31.027763) -> (-19.906244, 29.377271)
  line L784 (-19.906244, 29.377271) -> (-20.967964, 27.898483)
  line L785 (-20.967964, 27.898483) -> (-21.249904, 27.366353)
  line L786 (-21.249904, 27.366353) -> (-21.531844, 26.835747)
  line L787 (-21.531844, 26.835747) -> (-22.166844, 25.130137)
  line L788 (-22.166844, 25.130137) -> (-22.603724, 22.825849)